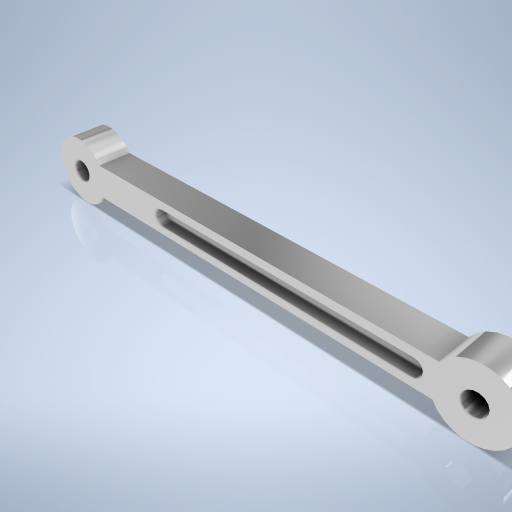
# Autodesk Inventor part: pleuel_third
Saved by Autodesk Inventor 2024.2 (Build 282272000, 272)
## iProperties
Created: 2024-05-05
Part Number: pleuel_third
Material: Nickel-Kupfer-Legierung 400
Document SubType Name: Modeling
Designer: Fabri
Density: 8.83 g/cm^3
Appearance: Chrom - poliert
Author: Fabri
Autodesk Inventor part; units mm, degrees
ref_plane "Arbeitsebene3" through (-142.5, 0, 0) normal (1, 0, 0) x (0, 1, 0)
sketch "Skizze1" plane through (0, 0, 0) normal (0, 1, 0) x (-1, 0, 0)
  arc A0 (10.3923, 6) -> (10.3923, -6) centre (0, 0) ccw
  line L0 (10.3923, 6) -> (150, 6)
  line L1 (150, 6) -> (150, -6)
  line L2 (150, -6) -> (10.3923, -6)
  line L3 (0, 0) -> (150, 0) construction
  circle A1 centre (0, 0) radius 3.75
  dimension "d0" = 24
  dimension "d1" = 12
  dimension "d2" = 7.5
  dimension "d3" = 150
  constraints: 8 end point, 2 centre point, 2 coincident, 2 horizontal, 2 point on circle, 1 midpoint, 1 parallel, 1 perpendicular, 1 other
  measures "d0" diameter of A0
  measures "d1" distance between parallel lines of L2 L0
  measures "d2" diameter of A1
  measures "d3" distance from line of point (0, 0) L1
extrude "Extrusion1" add sketch "Skizze1" along normal mid plane 12
ref_plane "Arbeitsebene1" through (0, 0, 0) normal (0, 1, 0) x (-1, 0, 0)
sketch "Skizze2" plane through (0, 0, 0) normal (0, 1, 0) x (-1, 0, 0)
  line L0 (150, 6) -> (150, -6) projected
  circle A0 centre (150, 0) radius 12
  point P0 (0, 0)
  dimension "d7" = 24
  constraints: 1 centre point, 1 midpoint
  measures "d7" diameter of A0
extrude "Extrusion2" add sketch "Skizze2" along normal mid plane 12
sketch "Skizze3" plane through (0, 6, 0) normal (0, 1, 0) x (1, 0, 0)
  arc A0 (-139.6077, 6) -> (-139.6077, -6) centre (-150, 0) ccw projected
  point P0 (0, 0)
  constraints: 1 coincident
hole "Bohrung1" at (-150, 6, 0) direction (0, -1, 0) diameter 7.5 depth 12
sketch "Skizze4" plane through (0, 6, 0) normal (0, 1, 0) x (1, 0, 0)
  line L0 (-17, 0) -> (-109, 0) construction
  line L1 (-17, 3) -> (-109, 3)
  line L2 (-109, -3) -> (-17, -3)
  arc A0 (-17, -3) -> (-17, 3) centre (-17, 0) ccw
  arc A1 (-109, 3) -> (-109, -3) centre (-109, 0) ccw
  circle A2 centre (-150, 0) radius 3.75 projected
  point P0 (0, 0)
  point P1 (-63, 0)
  point P2 (-14, 0)
  point P3 (-112, 0)
  point P4 (-63, 3)
  dimension "d18" = 6
  dimension "d20" = 98
  dimension "d21" = 150
  dimension "d22" = 14
  constraints: 8 end point, 6 point on circle, 4 tangent, 2 centre point, 2 midpoint, 1 horizontal, 1 horizontal alignment, 1 parallel, 1 vertical alignment
  measures "d18" distance between parallel lines of L1 L2
  measures "d20" distance of point (-14, 0) point (-112, 0)
  measures "d21" distance of point (0, 0) A2.centre
  measures "d22" distance of point (0, 0) point (-14, 0)
extrude "Extrusion3" cut sketch "Skizze4" against normal blind 4 contours A0 L2 A1 L1
mirror "Spiegeln1" about plane through (0, 0, 0) normal (0, 1, 0) of "Extrusion3"
ref_plane "Arbeitsebene2" through (12, 0, 0) normal (1, 0, 0) x (0, 1, 0)
sketch "Skizze5" plane through (12, 0, 0) normal (1, 0, 0) x (0, 1, 0)
  point P0 (0, 0)
  point P1 (0, 0)
  constraints: 1 coincident
sketch "Skizze6" plane through (-142.5, 0, 0) normal (1, 0, 0) x (0, 1, 0)
  point P0 (0, 0)
  point P1 (0, 0)
  constraints: 1 coincident
